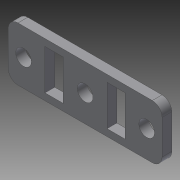
# Autodesk Inventor part: Vertical_Lead_Screw_E-stop_Plate
Saved by Autodesk Inventor 2015 (Build 190159000, 159)
## iProperties
Created: 2015-01-06
Part Number: Vertical_Lead_Screw_E-stop_Plate
Material: Generic
Document SubType Name: Modeling
Designer: Drew
Density: 1 g/cm^3
Appearance: Default
Author: Drew
Autodesk Inventor part; units mm, degrees
ref_plane "YZ Plane" through (0, 0, 0) normal (1, 0, 0) x (0, 1, 0)
ref_plane "XZ Plane" through (0, 0, 0) normal (0, 1, 0) x (-1, 0, 0)
ref_plane "XY Plane" through (0, 0, 0) normal (0, 0, 1) x (1, 0, 0)
sketch "Sketch1" plane through (0, 0, 0) normal (0, 0, 1) x (1, 0, 0)
  line L0 (43.65, -17.5) -> (-43.65, -17.5)
  line L1 (-50, -11.15) -> (-50, 11.15)
  line L2 (-43.65, 17.5) -> (43.65, 17.5)
  line L3 (50, 11.15) -> (50, -11.15)
  line L4 (50, -17.5) -> (-50, 17.5) construction
  line L5 (-50, -17.5) -> (50, 17.5) construction
  line L6 (0, 51.2558) -> (0, -45.9758)
  circle A0 centre (-40, 0) radius 5.1
  line L7 (-83.6339, 0) -> (65.0593, 0)
  circle A1 centre (40, 0) radius 5.1
  circle A2 centre (0, 0) radius 5.1
  arc A3 (-43.65, 17.5) -> (-50, 11.15) centre (-43.65, 11.15) ccw
  arc A4 (-50, -11.15) -> (-43.65, -17.5) centre (-43.65, -11.15) ccw
  arc A5 (43.65, -17.5) -> (50, -11.15) centre (43.65, -11.15) ccw
  arc A6 (50, 11.15) -> (43.65, 17.5) centre (43.65, 11.15) ccw
  line L8 (-14.2247, -13.0464) -> (-26.0744, -13.0464)
  line L9 (-26.0744, -13.0464) -> (-26.0744, 13.0464)
  line L10 (-26.0744, 13.0464) -> (-14.2247, 13.0464)
  line L11 (-14.2247, 13.0464) -> (-14.2247, -13.0464)
  line L12 (-14.2247, -13.0464) -> (-26.0744, 13.0464) construction
  line L13 (-26.0744, -13.0464) -> (-14.2247, 13.0464) construction
  line L14 (14.2247, -13.0464) -> (26.0744, -13.0464)
  line L15 (26.0744, -13.0464) -> (26.0744, 13.0464)
  line L16 (26.0744, 13.0464) -> (14.2247, 13.0464)
  line L17 (14.2247, 13.0464) -> (14.2247, -13.0464)
  line L18 (14.2247, -13.0464) -> (26.0744, 13.0464) construction
  line L19 (26.0744, -13.0464) -> (14.2247, 13.0464) construction
  point P0 (0, 0)
  point P1 (0, 0)
  point P2 (-20.1495, 0)
  point P3 (20.1495, 0)
  dimension "d0" = 100
  dimension "d1" = 35
  dimension "d2" = 80
  dimension "d3" = 10.2
  dimension "d6" = 10.2
  dimension "d7" = 6.35
  dimension "d8" = 26.0929
  dimension "d9" = 11.8497
  constraints: 40 end point, 12 point on line, 8 midpoint, 8 point on circle, 8 tangent, 7 centre point, 6 symmetric about line, 4 parallel, 3 equal radius, 3 horizontal, 2 perpendicular, 1 coincident, 1 vertical, 1 other
  measures "d0" distance of L4.end L5.end
  measures "d1" distance of L5.start L4.end
  measures "d2" diameter of A0.centre L6
  measures "d3" diameter of A0
  measures "d6" diameter of A2
  measures "d7" radius of A3
  measures "d8" distance of L8.end L9.end
  measures "d9" distance of L9.end L10.end
extrude "Extrusion1" add sketch "Sketch1" along normal blind 6.35 contours L0 L6 A2 L7 L17 L14 L15 A1 L3 A5 | L0 A4 L1 L7 A0 L9 L8 L11 A2 L6 | L7 A1 L15 L16 L17 A2 L6 L2 A6 L3 | L7 L11 L10 L9 A0 L1 A3 L2 L6 A2
equation "\"d6\" = d3"
body "Solid1"
